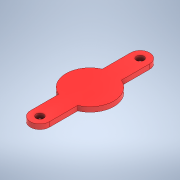
# Autodesk Inventor part: EslabonTransmisor
Saved by Autodesk Inventor 2021 (Build 250183000, 183)
## iProperties
Created: 2022-11-01
Part Number: EslabonTransmisor
Material: Generic
Document SubType Name: Modeling
Designer: USUARIO
Density: 1 g/cm^3
Appearance: Light Red
Author: USUARIO
Autodesk Inventor part; units mm, degrees
ref_plane "YZ Plane" through (0, 0, 0) normal (1, 0, 0) x (0, 1, 0)
ref_plane "XZ Plane" through (0, 0, 0) normal (0, 1, 0) x (-1, 0, 0)
ref_plane "XY Plane" through (0, 0, 0) normal (0, 0, 1) x (1, 0, 0)
sketch "Sketch1" plane through (0, 0, 0) normal (0, 1, 0) x (-1, 0, 0)
  line L0 (0, 52.5) -> (0, -52.5) construction
  line L1 (-10, 52.5) -> (-10, -52.5)
  line L2 (10, -52.5) -> (10, 52.5)
  arc A0 (10, 52.5) -> (-10, 52.5) centre (0, 52.5) ccw
  arc A1 (-10, -52.5) -> (10, -52.5) centre (0, -52.5) ccw
  circle A2 centre (0, 0) radius 25
  line L3 (35, 0) -> (-35, 0) projected
  circle A3 centre (0, 52.5) radius 4
  circle A4 centre (0, -52.5) radius 4
  line L4 (0, -87.5) -> (0, 87.5) projected
  point P0 (10, -22.9129)
  point P1 (10, 22.9129)
  point P2 (-10, 22.9129)
  point P3 (-10, -22.9129)
  dimension "d0" = 50
  dimension "d1" = 8
  dimension "d2" = 8
  dimension "d3" = 20
  dimension "d4" = 105
  constraints: 8 end point, 5 centre point, 4 point on circle, 4 tangent, 3 coincident, 3 midpoint, 1 parallel, 1 vertical
  measures "d0" diameter of A2
  measures "d1" diameter of A3
  measures "d2" diameter of A4
  measures "d3" distance between parallel lines of L1 L2
  measures "d4" distance of L2.start L2.end
extrude "Extrusion1" add sketch "Sketch1" along normal blind 5 contours A0 L4 A3 A2 L1 | A2 L4 L3 L1 | L1 L3 A2 | A0 L2 A2 L4 A3 | L3 L4 A2 L1 | L1 A2 L3 | A2 L2 L3 L4 | A2 L4 A4 A1 L1 | L3 L2 A2 L4 | A2 L3 L2 | A2 L2 A1 L4 A4 | L3 A2 L2
equation "\"d0\" = DV"
equation "\"d3\" = AnEsl"
equation "\"DV\" = 50"
equation "\"AnEsl\" = 20"
body "Solid1"
